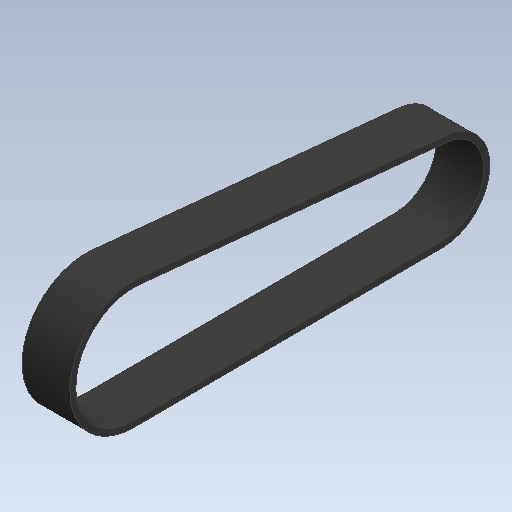
# Autodesk Inventor part: remen
Saved by Autodesk Inventor 2020 (Build 240168000, 168)
## iProperties
Created: 2024-02-27
Part Number: remen
Material: Типовые
Document SubType Name: Modeling
Designer: 4s
Density: 1 g/cm^3
Appearance: Резина — черная
Author: 4s
Autodesk Inventor part; units mm, degrees
ref_plane "YZ Plane" through (0, 0, 0) normal (1, 0, 0) x (0, 1, 0)
ref_plane "XZ Plane" through (0, 0, 0) normal (0, 1, 0) x (-1, 0, 0)
ref_plane "XY Plane" through (0, 0, 0) normal (0, 0, 1) x (1, 0, 0)
sketch "Эскиз1" plane through (0, 0, 0) normal (1, 0, 0) x (0, 1, 0)
  arc A0 (7.9613, -0.7862) -> (-7.9999, -0.0361) centre (0, 0) ccw
  arc A1 (-7.8247, -38.8562) -> (4.1462, -39.4188) centre (-1.8248, -38.8291) ccw
  line L0 (7.9613, -0.7862) -> (4.1462, -39.4188)
  line L1 (-7.9999, -0.0361) -> (-7.8247, -38.8562)
  arc A2 (-7.9999, -0.0361) -> (7.9613, -0.7862) centre (0, 0) ccw construction
  arc A3 (4.1462, -39.4188) -> (-7.8247, -38.8562) centre (-1.8248, -38.8291) ccw construction
  arc A4 (7.2149, -0.7125) -> (-7.2499, -0.0327) centre (0, 0) ccw
  arc A5 (-7.0747, -38.8528) -> (3.3998, -39.3451) centre (-1.8248, -38.8291) ccw
  line L2 (7.2149, -0.7125) -> (3.3998, -39.3451)
  line L3 (0, 0) -> (-1.8248, -38.8291) construction
  line L4 (-7.2499, -0.0327) -> (-7.0747, -38.8528)
  arc A6 (-1.5783, -33.5849) -> (-7.0747, -38.8528) centre (-1.8248, -38.8291) ccw construction
  arc A7 (3.3998, -39.3451) -> (-1.5783, -33.5849) centre (-1.8248, -38.8291) ccw construction
  arc A8 (-0.3403, -7.242) -> (7.2149, -0.7125) centre (0, 0) ccw construction
  arc A9 (-7.2499, -0.0327) -> (-0.3403, -7.242) centre (0, 0) ccw construction
  dimension "d0" = 38.872
  dimension "d1" = 16
  dimension "d2" = 12
  dimension "d3" = 14.5
  dimension "d4" = 10.5
  constraints: 20 point on circle, 10 centre point, 10 end point, 8 tangent, 3 coincident, 2 point on line, 2 symmetric about line
  measures "d0" distance of point (0, 0) A1.centre
  measures "d1" diameter of A0
  measures "d2" diameter of A1
  measures "d3" diameter of A4
  measures "d4" diameter of A5
extrude "Выдавливание1" add sketch "Эскиз1" along normal blind 6
